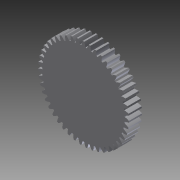
# Autodesk Inventor part: Part6
Saved by Autodesk Inventor 2012 (Build 160160000, 160)
## iProperties
Created: 2013-11-18
Part Number: Part6
Material: Default
Document SubType Name: Modeling
Designer: fqian3
Density: 1 g/cm^3
Author: fqian3
Autodesk Inventor part; units mm, degrees
ref_plane "YZ Plane" through (0, 0, 0) normal (1, 0, 0) x (0, 1, 0)
ref_plane "XZ Plane" through (0, 0, 0) normal (0, 1, 0) x (-1, 0, 0)
ref_plane "XY Plane" through (0, 0, 0) normal (0, 0, 1) x (1, 0, 0)
sketch "Sketch1" plane through (0, 0, 0) normal (0, 0, 1) x (1, 0, 0)
  circle A0 centre (0, 0) radius 25.4
  dimension "d0" = 50.8
  constraints: 1 centre point, 1 coincident
  measures "d0" diameter of A0
extrude "Extrusion1" add sketch "Sketch1" along normal blind 6.35
spur gear teeth "Spur Gear2" teeth 47 pitch diameter 42.6357 tip diameter 44.0431 root diameter 39.9609 face width 6.35 trims to tip circle yes start plane through (0, 0, 6.35) normal (0, 0, 1) x (1, 0, 0)
body "Solid1"
